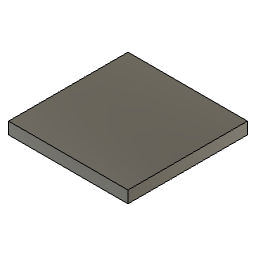
Meltybrain CAD v0.3 v24 (Autodesk Fusion 360 archive; units mm, degrees)
design "Accelerometer Model"
Autodesk Fusion 360 part; units mm, degrees
sketch "Sketch1" plane through (0, 0, 0) normal (0, 0, 1) x (1, 0, 0)
  line L0 (0, 0) -> (0, 20)
  line L1 (0, 20) -> (20, 20)
  line L2 (20, 20) -> (20, 0)
  line L3 (20, 0) -> (0, 0)
  dimension "d2" = 20
  dimension "d3" = 20
  dimension "d4" = 20
  constraint coincident L0.start L3.end
  constraint vertical L0
  constraint perpendicular L0 L1
  constraint perpendicular L1 L2
  measures "d2" distance of L0.start L0.end
  measures "d3" distance of L0.end L1.end
  measures "d4" distance of L1.end L2.end
extrude "Extrude1" add sketch "Sketch1" along normal blind 2

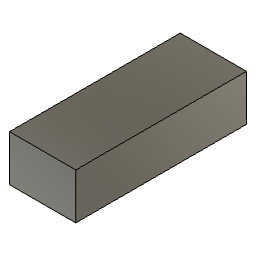
design "GNB 4s 530mAh Model"
Autodesk Fusion 360 part; units mm, degrees
sketch "Sketch1" plane through (0, 0, 0) normal (0, 0, 1) x (1, 0, 0)
  line L0 (0, 0) -> (0, 67)
  line L1 (0, 67) -> (26, 67)
  line L2 (26, 67) -> (26, 0)
  line L3 (26, 0) -> (0, 0)
  dimension "d1" = 67
  dimension "d2" = 26
  dimension "d3" = 67
  constraint coincident L0.start L3.end
  constraint vertical L0
  constraint perpendicular L0 L1
  constraint perpendicular L1 L2
  measures "d1" distance of L0.start L0.end
  measures "d2" distance of L0.end L1.end
  measures "d3" distance of L1.end L2.end
extrude "Extrude1" add sketch "Sketch1" along normal blind 18

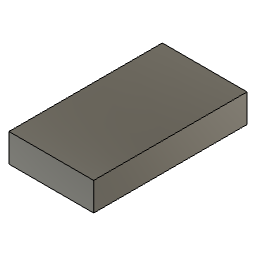
design "ESC Model"
Autodesk Fusion 360 part; units mm, degrees
sketch "Sketch1" plane through (0, 0, 0) normal (0, 0, 1) x (1, 0, 0)
  line L0 (0, 0) -> (0, 38)
  line L1 (0, 38) -> (21, 38)
  line L2 (21, 38) -> (21, 0)
  line L3 (21, 0) -> (0, 0)
  dimension "d1" = 38
  dimension "d2" = 21
  dimension "d3" = 38
  constraint coincident L0.start L3.end
  constraint vertical L0
  constraint perpendicular L0 L1
  constraint perpendicular L1 L2
  measures "d1" distance of L0.start L0.end
  measures "d2" distance of L0.end L1.end
  measures "d3" distance of L1.end L2.end
extrude "Extrude1" add sketch "Sketch1" along normal blind 7
